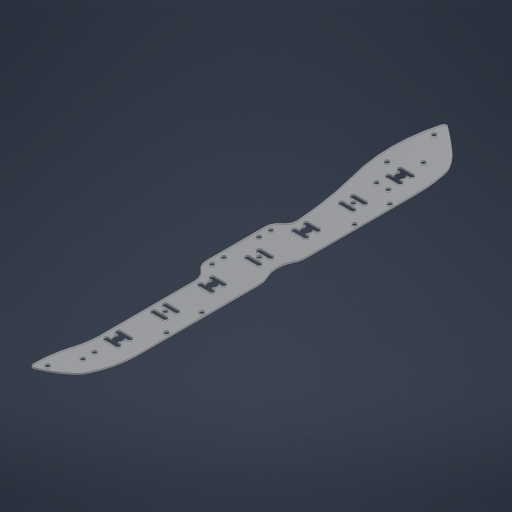
# Autodesk Inventor part: sled2
Saved by Autodesk Inventor 2024 (Build 280153000, 153)
## iProperties
Created: 2023-10-30
Part Number: sled2
Material: Polycarbonate, Smoke
Document SubType Name: Modeling
Designer: macbook
Density: 1.2 g/cm^3
Appearance: Polycarbonate - Clear(1)
Author: macbook
Autodesk Inventor part; units mm, degrees
ref_plane "YZ Plane" through (0, 0, 0) normal (1, 0, 0) x (0, 1, 0)
ref_plane "XZ Plane" through (0, 0, 0) normal (0, 1, 0) x (-1, 0, 0)
ref_plane "XY Plane" through (0, 0, 0) normal (0, 0, 1) x (1, 0, 0)
sketch "Sketch2" plane through (0, 0, 0) normal (0, 1, 0) x (-1, 0, 0)
  line L0 (25.3485, -88.9331) -> (25.3485, -76.2331)
  line L1 (25.3485, -76.2331) -> (0.0063, -76.2331)
  line L2 (0.0063, -76.2331) -> (0.0055, -63.5331)
  line L3 (0.1328, -20.6833) -> (0.1265, -35.8822)
  line L4 (38.2012, -93.5899) -> (38.2012, -99.9399)
  line L5 (12.8495, -23.9499) -> (19.1995, -23.9501)
  line L6 (19.1995, -23.9501) -> (6.4995, -23.9497)
  line L7 (25.3485, -88.9331) -> (31.6373, -88.0533)
  arc A0 (30.6963, -113.4359) -> (33.2246, -115.3327) centre (248.7957, 174.6442) ccw
  line L8 (38.2825, -88.8911) -> (38.2774, -69.8411)
  line L9 (38.2774, -69.8411) -> (44.78, -69.8393)
  arc A1 (38.3114, -113.5855) -> (38.3007, -17.4758) centre (-135.3855, -65.5498) ccw
  arc A2 (33.2246, -115.3327) -> (38.3114, -113.5855) centre (35.1695, -112.7166) ccw
  arc A3 (44.8311, -65.5299) -> (38.2642, -32.0968) centre (-43.6087, -65.5397) ccw
  line L10 (6.4995, -23.9497) -> (0.1314, -23.947)
  line L11 (0.1314, -23.947) -> (0.2658, 299.9029) construction
  line L12 (0.2658, 299.9029) -> (25.6658, 299.9029) construction
  line L13 (25.6658, 269.4446) -> (25.6658, -23.6933)
  line L14 (25.6658, -23.6933) -> (39.903, -23.6933)
  line L15 (0.2658, 299.9029) -> (-12.4342, 299.9029)
  line L16 (-12.5436, -23.9601) -> (-12.5436, -35.112)
  arc A4 (-4.3142, -80.5045) -> (7.2064, -94.0414) centre (51.9465, -44.2947) ccw
  arc A5 (-12.5436, -35.112) -> (-9.0134, -68.7415) centre (149.4014, -35.112) ccw
  arc A6 (-5.9833, -77.5413) -> (-4.3142, -80.5045) centre (19.9766, -64.8707) ccw
  arc A7 (-9.0134, -68.7415) -> (-5.9833, -77.5413) centre (28.2561, -60.8297) ccw
  arc A8 (7.2064, -94.0414) -> (30.6963, -113.4359) centre (248.7971, 174.6431) ccw
  line L17 (0.2658, 299.9029) -> (0.1867, 109.403) construction
  line L18 (0.1867, 109.403) -> (-36.5163, 109.4182)
  arc A9 (-9.714, 95.5829) -> (-9.702, 123.2303) centre (-36.5163, 109.4182) ccw
  line L19 (-12.5217, 258.1981) -> (-12.5217, 134.8616)
  line L20 (-12.5436, 83.9322) -> (-12.5436, -23.9601)
  arc A10 (-12.5217, 127.6948) -> (-12.5436, 91.1127) centre (-36.5163, 109.4182) ccw construction
  arc A11 (-12.5217, 134.8616) -> (-9.702, 123.2303) centre (12.8783, 134.8616) ccw
  arc A12 (-9.714, 95.5829) -> (-12.5436, 83.9322) centre (12.8564, 83.9322) ccw
  line L21 (25.6658, 299.9029) -> (25.6658, 331.6529)
  line L22 (25.6658, 331.6529) -> (32.0158, 331.6529)
  arc A13 (35.1908, 331.6395) -> (28.8408, 331.6529) centre (32.0158, 331.6529) ccw
  line L23 (0.2658, 299.9029) -> (0.2658, 325.3029)
  line L24 (32.0158, 331.6529) -> (30.6929, 331.6529)
  arc A14 (29.2214, 292.4497) -> (35.1908, 331.6395) centre (-92.7618, 331.0796) ccw
  line L25 (31.9383, 334.827) -> (31.4142, 334.827)
  arc A15 (31.007, 334.6634) -> (4.0007, 318.3551) centre (65.1249, 247.6497) ccw
  arc A16 (-10.3215, 302.8155) -> (-14.0041, 295.5815) centre (10.1821, 287.8234) ccw
  line L26 (-12.5217, 258.1981) -> (-12.5217, 338.0406)
  arc A17 (-2.1991, 310.3119) -> (-12.5217, 265.7661) centre (88.7553, 265.7661) ccw
  arc A18 (4.0007, 318.3551) -> (-2.1991, 310.3119) centre (20.612, 299.1399) ccw
  line L27 (0.2658, 299.9029) -> (0.2605, 287.2029)
  line L28 (0.2605, 287.2029) -> (12.9605, 287.1977)
  line L29 (0.1867, 109.403) -> (0.221, 191.953)
  line L30 (0.221, 191.953) -> (-7.7165, 191.9562)
  line L31 (0.1867, 109.403) -> (0.1525, 26.853)
  line L32 (0.1525, 26.853) -> (-7.785, 26.853)
  line L33 (-7.785, 26.853) -> (-7.785, -11.247)
  line L34 (-7.7165, 191.9562) -> (-7.7165, 230.0562)
  arc A19 (25.6658, 282.6329) -> (27.2405, 286.6766) centre (-92.7618, 331.0796) ccw
  arc A20 (29.2214, 292.4497) -> (25.6658, 269.4446) centre (101.8658, 269.4446) ccw
  line L35 (25.6658, 109.403) -> (32.0158, 109.403)
  line L36 (32.0158, 109.403) -> (32.0158, 90.353)
  line L37 (32.0158, 90.353) -> (32.0158, 77.653)
  line L38 (32.0158, 109.403) -> (32.0158, 128.453)
  line L39 (32.0158, 128.453) -> (32.0158, 141.153)
  line L40 (32.0158, 109.403) -> (38.3658, 109.403)
  line L41 (38.3658, 109.403) -> (38.3658, 141.153)
  arc A21 (38.3658, 141.153) -> (32.0778, 153.6114) centre (22.8798, 141.153) ccw
  arc A22 (25.6658, 83.9658) -> (25.6658, 78.268) centre (416.3302, 81.1169) ccw
  arc A23 (26.6118, 53.7976) -> (38.3007, -17.4758) centre (416.3302, 81.1169) ccw
  arc A24 (25.6658, 166.3155) -> (32.0778, 153.6114) centre (41.457, 166.3155) ccw
  line L42 (38.3658, 109.403) -> (38.3658, 77.653)
  arc A25 (32.0778, 65.1945) -> (38.3658, 77.653) centre (22.8798, 77.653) ccw
  arc A26 (32.0778, 65.1945) -> (30.3394, 63.7048) centre (41.457, 52.4904) ccw
  arc A27 (30.3394, 63.7048) -> (26.6118, 53.7976) centre (39.2807, 54.6857) ccw
  line L43 (25.6658, 299.9029) -> (25.6658, 325.3029)
  line L44 (12.9605, 287.1977) -> (12.9605, 299.8977)
  point P0 (0.0775, -39.6857)
  point P1 (12.8012, -68.1967)
  point P2 (37.0807, -118.1599)
  point P3 (33.0954, -49.1463)
  point P4 (33.0954, -99.9463)
  point P5 (33.0954, -99.9463)
  point P6 (33.0954, -49.1463)
  point P7 (30.6993, 334.5421)
  point P8 (25.6658, 160.9899)
  point P9 (25.6658, 57.8161)
  point P10 (25.6658, 52.4904)
  point P11 (26.3876, 57.21)
  dimension "d3" = 12.7
  dimension "d5" = 12.7
  dimension "d37" = 6.35
  dimension "d54" = 6.35
  dimension "d55" = 25.4
  dimension "d58" = 19.05
  dimension "d82" = 323.85
  dimension "d83" = 25.4
  dimension "d84" = 12.7
  dimension "d85" = 38.1
  dimension "d86" = 190.5
  dimension "d87" = 60.325
  dimension "d88" = 36.703
  dimension "d89" = 25.4
  dimension "d93" = 6.35
  dimension "d94" = 6.35
  dimension "d95" = 31.75
  dimension "d97" = 25.4
  dimension "d99" = 25.4
  dimension "d102" = 25.4
  dimension "d103" = 12.7
  dimension "d104" = 12.7
  dimension "d105" = 82.55
  dimension "d106" = 7.9375
  dimension "d107" = 82.55
  dimension "d108" = 38.1
  dimension "d109" = 38.1
  dimension "d110" = 76.2
  dimension "d111" = 6.35
  dimension "d112" = 19.05
  dimension "d113" = 12.7
  dimension "d114" = 19.05
  dimension "d115" = 12.7
  dimension "d116" = 6.35
  dimension "d117" = 31.75
  dimension "d118" = 12.7
  dimension "d119" = 12.7
  constraints: 90 end point, 67 point on circle, 28 centre point, 22 tangent, 21 point on line, 18 coincident, 13 perpendicular, 10 vertical, 6 horizontal, 5 symmetric about line, 1 equal radius, 1 midpoint, 2 other
  measures "d3" distance of L0.start L0.end
  measures "d5" distance of L1.end L2.end
  measures "d37" distance of L5.start L5.end
  measures "d54" distance of L0.start L7.end
  measures "d55" distance of L7.end A0.start
  measures "d58" distance of L8.start L8.end
  measures "d82" distance of L10.end L11.end
  measures "d83" distance of L11.end L12.end
  measures "d84" distance of L11.end L15.end
  measures "d85" radius of A7
  measures "d86" distance of L11.end L17.end
  measures "d87" diameter of A9
  measures "d88" distance of L17.end L18.end
  measures "d89" radius of A11
  measures "d93" distance of L21.end L22.end
  measures "d94" diameter of A13
  measures "d95" distance of L12.end L21.end
  measures "d97" distance of L11.end L23.end
  measures "d99" radius of A16
  measures "d102" radius of A18
  measures "d103" distance of L11.end L27.end
  measures "d104" distance of L27.end L28.end
  measures "d105" distance of L17.end L29.end
  measures "d106" distance of L29.end L30.end
  measures "d107" distance of L17.end L31.end
  measures "d108" distance of L33.start L33.end
  measures "d109" distance of L34.start L34.end
  measures "d110" radius of A20
  measures "d111" distance of L35.start L35.end
  measures "d112" distance of L35.end L36.end
  measures "d113" distance of L36.end L37.end
  measures "d114" distance of L35.end L38.end
  measures "d115" distance of L38.end L39.end
  measures "d116" distance of L40.start L40.end
  measures "d117" distance of L40.end L41.end
  measures "d118" radius of A27
  measures "d119" distance of L44.start L44.end
extrude "Extrusion1" add sketch "Sketch2" along normal blind 1.5875 contours A8 A4 A6 A7 A5 L16 L20 A12 A9 A11 L19 L26 A17 L15 L23 A18 A15 A13 A14 A20 L13 A22 L14 A1 A2 A0 | L14 L13 L35 L40 L42 A25 A26 A27 A23 A1 | A22 L13 | L13 A24 A21 L41 L40 L35 | A17 A18 L23 L15 | A15 A13
hole "Hole3" at (-6.4995, 0, -23.9497) at (-19.1995, 0, -23.9501) at (-12.8012, 0, -68.1967) at (-33.0954, 0, -49.1463) at (-33.0954, 0, -99.9463) at (-12.9605, 0, 287.1977) at (7.7165, 0, 191.9562) at (7.785, 0, 26.853) at (7.785, 0, -11.247) at (7.7165, 0, 230.0562) at (-32.0158, 0, 141.153) at (-32.0158, 0, 128.453) at (-32.0158, 0, 90.353) at (-32.0158, 0, 77.653) at (-25.6658, 0, 325.3029) at (-12.9605, 0, 299.8977) direction (0, 1, 0) diameter 4.7625 end through all
sketch "Sketch4" plane through (0, 1.5875, 0) normal (0, 1, 0) x (1, 0, 0)
  line L0 (-19.1995, 23.9497) -> (-19.1995, 42.9997) construction
  line L1 (-19.1995, 23.9497) -> (-0.1495, 23.9497) construction
  line L2 (-19.1995, 42.9997) -> (-12.8495, 42.9997)
  line L3 (-6.4995, 23.9497) -> (-6.4995, 36.6497) construction
  line L4 (-6.4995, 36.6497) -> (-19.1995, 36.6497) construction
  arc A0 (-19.1995, 39.0309) -> (-19.1995, 34.2684) centre (-19.1995, 36.6497) ccw
  arc A1 (-6.4995, 34.2684) -> (-6.4995, 39.0309) centre (-6.4995, 36.6497) ccw
  line L5 (-19.1995, 34.2684) -> (-6.4995, 34.2684)
  line L6 (-6.4995, 36.6497) -> (-6.4995, 49.3497) construction
  line L7 (-6.4995, 49.3497) -> (-19.1995, 49.3497) construction
  arc A2 (-19.1995, 51.7309) -> (-19.1995, 46.9684) centre (-19.1995, 49.3497) ccw
  arc A3 (-6.4995, 46.9684) -> (-6.4995, 51.7309) centre (-6.4995, 49.3497) ccw
  line L8 (-6.4995, 51.7309) -> (-19.1995, 51.7309)
  line L9 (-12.8495, 34.2684) -> (-12.8495, 36.6497)
  line L10 (-12.8495, 36.6497) -> (-19.1995, 36.6497)
  line L11 (-19.1995, 39.0309) -> (-16.0205, 39.0309)
  line L12 (-6.4995, 39.0309) -> (-9.6785, 39.0309)
  line L13 (-6.4995, 46.9684) -> (-9.2483, 46.9684)
  line L14 (-19.1995, 46.9684) -> (-16.4508, 46.9684)
  arc A4 (-9.8454, 39.5008) -> (-9.4379, 46.5192) centre (-12.8495, 43.1963) ccw
  arc A5 (-16.2612, 46.5192) -> (-15.8536, 39.5008) centre (-12.8495, 43.1963) ccw
  arc A6 (-9.8454, 39.5008) -> (-9.6785, 39.0309) centre (-9.6785, 39.2955) ccw
  arc A7 (-16.0205, 39.0309) -> (-15.8536, 39.5008) centre (-16.0205, 39.2955) ccw
  arc A8 (-16.2612, 46.5192) -> (-16.4508, 46.9684) centre (-16.4508, 46.7038) ccw
  arc A9 (-9.2483, 46.9684) -> (-9.4379, 46.5192) centre (-9.2483, 46.7038) ccw
  line L15 (-6.4995, 23.9497) -> (-12.8495, 23.9497) construction
  line L16 (-12.8495, 23.9497) -> (-12.8495, -77.6503) construction
  line L17 (-12.8495, -77.6503) -> (-12.8495, -179.2503) construction
  line L18 (-12.8495, -179.2503) -> (-12.8495, -280.8503) construction
  arc A10 (-19.1995, -49.8691) -> (-19.1995, -54.6316) centre (-19.1995, -52.2503) ccw
  arc A11 (-6.4995, -67.3316) -> (-6.4995, -62.5691) centre (-6.4995, -64.9503) ccw
  arc A12 (-6.4995, -54.6316) -> (-6.4995, -49.8691) centre (-6.4995, -52.2503) ccw
  line L19 (-6.4995, -54.6316) -> (-9.2483, -54.6316)
  line L20 (-19.1995, -54.6316) -> (-16.4508, -54.6316)
  arc A13 (-16.2612, -55.0808) -> (-16.4508, -54.6316) centre (-16.4508, -54.8962) ccw
  line L21 (-19.1995, -58.6003) -> (-12.8495, -58.6003)
  line L22 (-6.4995, -49.8691) -> (-19.1995, -49.8691)
  arc A14 (-9.2483, -54.6316) -> (-9.4379, -55.0808) centre (-9.2483, -54.8962) ccw
  arc A15 (-16.2612, -55.0808) -> (-15.8536, -62.0992) centre (-12.8495, -58.4037) ccw
  line L23 (-6.4995, -52.2503) -> (-19.1995, -52.2503) construction
  arc A16 (-9.8454, -62.0992) -> (-9.4379, -55.0808) centre (-12.8495, -58.4037) ccw
  line L24 (-6.4995, -64.9503) -> (-6.4995, -52.2503) construction
  arc A17 (-19.1995, -62.5691) -> (-19.1995, -67.3316) centre (-19.1995, -64.9503) ccw
  line L25 (-6.4995, -64.9503) -> (-19.1995, -64.9503) construction
  line L26 (-19.1995, -67.3316) -> (-6.4995, -67.3316)
  line L27 (-19.1995, -62.5691) -> (-16.0205, -62.5691)
  arc A18 (-16.0205, -62.5691) -> (-15.8536, -62.0992) centre (-16.0205, -62.3045) ccw
  line L28 (-12.8495, -64.9503) -> (-19.1995, -64.9503)
  arc A19 (-9.8454, -62.0992) -> (-9.6785, -62.5691) centre (-9.6785, -62.3045) ccw
  line L29 (-6.4995, -62.5691) -> (-9.6785, -62.5691)
  line L30 (-12.8495, -67.3316) -> (-12.8495, -64.9503)
  arc A20 (-19.1995, -151.4691) -> (-19.1995, -156.2316) centre (-19.1995, -153.8503) ccw
  arc A21 (-6.4995, -168.9316) -> (-6.4995, -164.1691) centre (-6.4995, -166.5503) ccw
  arc A22 (-6.4995, -156.2316) -> (-6.4995, -151.4691) centre (-6.4995, -153.8503) ccw
  line L31 (-6.4995, -156.2316) -> (-9.2483, -156.2316)
  line L32 (-19.1995, -156.2316) -> (-16.4508, -156.2316)
  arc A23 (-16.2612, -156.6808) -> (-16.4508, -156.2316) centre (-16.4508, -156.4962) ccw
  line L33 (-19.1995, -160.2003) -> (-12.8495, -160.2003)
  line L34 (-6.4995, -151.4691) -> (-19.1995, -151.4691)
  arc A24 (-9.2483, -156.2316) -> (-9.4379, -156.6808) centre (-9.2483, -156.4962) ccw
  arc A25 (-16.2612, -156.6808) -> (-15.8536, -163.6992) centre (-12.8495, -160.0037) ccw
  line L35 (-6.4995, -153.8503) -> (-19.1995, -153.8503) construction
  arc A26 (-9.8454, -163.6992) -> (-9.4379, -156.6808) centre (-12.8495, -160.0037) ccw
  line L36 (-6.4995, -166.5503) -> (-6.4995, -153.8503) construction
  arc A27 (-19.1995, -164.1691) -> (-19.1995, -168.9316) centre (-19.1995, -166.5503) ccw
  line L37 (-6.4995, -166.5503) -> (-19.1995, -166.5503) construction
  line L38 (-19.1995, -168.9316) -> (-6.4995, -168.9316)
  line L39 (-19.1995, -164.1691) -> (-16.0205, -164.1691)
  arc A28 (-16.0205, -164.1691) -> (-15.8536, -163.6992) centre (-16.0205, -163.9045) ccw
  line L40 (-12.8495, -166.5503) -> (-19.1995, -166.5503)
  arc A29 (-9.8454, -163.6992) -> (-9.6785, -164.1691) centre (-9.6785, -163.9045) ccw
  line L41 (-6.4995, -164.1691) -> (-9.6785, -164.1691)
  line L42 (-12.8495, -168.9316) -> (-12.8495, -166.5503)
  arc A30 (-19.1995, -253.0691) -> (-19.1995, -257.8316) centre (-19.1995, -255.4503) ccw
  arc A31 (-6.4995, -270.5316) -> (-6.4995, -265.7691) centre (-6.4995, -268.1503) ccw
  arc A32 (-6.4995, -257.8316) -> (-6.4995, -253.0691) centre (-6.4995, -255.4503) ccw
  line L43 (-6.4995, -257.8316) -> (-9.2483, -257.8316)
  line L44 (-19.1995, -257.8316) -> (-16.4508, -257.8316)
  arc A33 (-16.2612, -258.2808) -> (-16.4508, -257.8316) centre (-16.4508, -258.0962) ccw
  line L45 (-19.1995, -261.8003) -> (-12.8495, -261.8003)
  line L46 (-6.4995, -253.0691) -> (-19.1995, -253.0691)
  arc A34 (-9.2483, -257.8316) -> (-9.4379, -258.2808) centre (-9.2483, -258.0962) ccw
  arc A35 (-16.2612, -258.2808) -> (-15.8536, -265.2992) centre (-12.8495, -261.6037) ccw
  line L47 (-6.4995, -255.4503) -> (-19.1995, -255.4503) construction
  arc A36 (-9.8454, -265.2992) -> (-9.4379, -258.2808) centre (-12.8495, -261.6037) ccw
  line L48 (-6.4995, -268.1503) -> (-6.4995, -255.4503) construction
  arc A37 (-19.1995, -265.7691) -> (-19.1995, -270.5316) centre (-19.1995, -268.1503) ccw
  line L49 (-6.4995, -268.1503) -> (-19.1995, -268.1503) construction
  line L50 (-19.1995, -270.5316) -> (-6.4995, -270.5316)
  line L51 (-19.1995, -265.7691) -> (-16.0205, -265.7691)
  arc A38 (-16.0205, -265.7691) -> (-15.8536, -265.2992) centre (-16.0205, -265.5045) ccw
  line L52 (-12.8495, -268.1503) -> (-19.1995, -268.1503)
  arc A39 (-9.8454, -265.2992) -> (-9.6785, -265.7691) centre (-9.6785, -265.5045) ccw
  line L53 (-6.4995, -265.7691) -> (-9.6785, -265.7691)
  line L54 (-12.8495, -270.5316) -> (-12.8495, -268.1503)
  line L55 (-12.8495, 23.9497) -> (-12.8495, -26.8503) construction
  arc A40 (-19.1995, 0.9309) -> (-19.1995, -3.8316) centre (-19.1995, -1.4503) ccw
  arc A41 (-6.4995, -16.5316) -> (-6.4995, -11.7691) centre (-6.4995, -14.1503) ccw
  arc A42 (-6.4995, -3.8316) -> (-6.4995, 0.9309) centre (-6.4995, -1.4503) ccw
  line L56 (-6.4995, -3.8316) -> (-9.2483, -3.8316)
  line L57 (-19.1995, -3.8316) -> (-16.4508, -3.8316)
  line L58 (-6.4995, 0.9309) -> (-19.1995, 0.9309)
  line L59 (-6.4995, -1.4503) -> (-19.1995, -1.4503) construction
  line L60 (-6.4995, -14.1503) -> (-6.4995, -1.4503) construction
  arc A43 (-19.1995, -11.7691) -> (-19.1995, -16.5316) centre (-19.1995, -14.1503) ccw
  line L61 (-6.4995, -14.1503) -> (-19.1995, -14.1503) construction
  line L62 (-19.1995, -16.5316) -> (-6.4995, -16.5316)
  line L63 (-19.1995, -11.7691) -> (-16.0205, -11.7691)
  line L64 (-12.8495, -14.1503) -> (-19.1995, -14.1503)
  line L65 (-6.4995, -11.7691) -> (-9.6785, -11.7691)
  line L66 (-12.8495, -16.5316) -> (-12.8495, -14.1503)
  circle A44 centre (-12.8495, -7.6037) radius 2.3812
  line L67 (-16.0205, -11.7691) -> (-9.6785, -11.7691)
  line L68 (-16.4508, -3.8316) -> (-9.2483, -3.8316)
  line L69 (-12.8495, -77.6503) -> (-12.8495, -128.4503)
  line L70 (-6.4995, -115.7503) -> (-6.4995, -103.0503) construction
  line L71 (-6.4995, -115.7503) -> (-19.1995, -115.7503) construction
  line L72 (-6.4995, -113.3691) -> (-9.6785, -113.3691)
  line L73 (-19.1995, -105.4316) -> (-16.4508, -105.4316)
  line L74 (-6.4995, -103.0503) -> (-19.1995, -103.0503) construction
  line L75 (-6.4995, -100.6691) -> (-19.1995, -100.6691)
  arc A45 (-19.1995, -100.6691) -> (-19.1995, -105.4316) centre (-19.1995, -103.0503) ccw
  line L76 (-12.8495, -115.7503) -> (-19.1995, -115.7503)
  line L77 (-19.1995, -113.3691) -> (-16.0205, -113.3691)
  line L78 (-6.4995, -105.4316) -> (-9.2483, -105.4316)
  arc A46 (-6.4995, -105.4316) -> (-6.4995, -100.6691) centre (-6.4995, -103.0503) ccw
  arc A47 (-6.4995, -118.1316) -> (-6.4995, -113.3691) centre (-6.4995, -115.7503) ccw
  arc A48 (-19.1995, -113.3691) -> (-19.1995, -118.1316) centre (-19.1995, -115.7503) ccw
  line L79 (-12.8495, -118.1316) -> (-12.8495, -115.7503)
  line L80 (-19.1995, -118.1316) -> (-6.4995, -118.1316)
  circle A49 centre (-12.8495, -109.2037) radius 2.3812
  line L81 (-16.0205, -113.3691) -> (-9.6785, -113.3691)
  line L82 (-16.4508, -105.4316) -> (-9.2483, -105.4316)
  line L83 (-12.8495, -179.2503) -> (-12.8495, -230.0503)
  arc A50 (-19.1995, -202.2691) -> (-19.1995, -207.0316) centre (-19.1995, -204.6503) ccw
  line L84 (-12.8495, -219.7316) -> (-12.8495, -217.3503)
  line L85 (-12.8495, -217.3503) -> (-19.1995, -217.3503)
  arc A51 (-19.1995, -214.9691) -> (-19.1995, -219.7316) centre (-19.1995, -217.3503) ccw
  line L86 (-6.4995, -217.3503) -> (-6.4995, -204.6503) construction
  circle A52 centre (-12.8495, -210.8037) radius 2.3812
  line L87 (-19.1995, -207.0316) -> (-16.4508, -207.0316)
  line L88 (-16.4508, -207.0316) -> (-9.2483, -207.0316)
  line L89 (-6.4995, -204.6503) -> (-19.1995, -204.6503) construction
  line L90 (-6.4995, -202.2691) -> (-19.1995, -202.2691)
  line L91 (-6.4995, -207.0316) -> (-9.2483, -207.0316)
  arc A53 (-6.4995, -207.0316) -> (-6.4995, -202.2691) centre (-6.4995, -204.6503) ccw
  line L92 (-6.4995, -214.9691) -> (-9.6785, -214.9691)
  arc A54 (-6.4995, -219.7316) -> (-6.4995, -214.9691) centre (-6.4995, -217.3503) ccw
  line L93 (-16.0205, -214.9691) -> (-9.6785, -214.9691)
  line L94 (-19.1995, -214.9691) -> (-16.0205, -214.9691)
  line L95 (-19.1995, -219.7316) -> (-6.4995, -219.7316)
  line L96 (-6.4995, -217.3503) -> (-19.1995, -217.3503) construction
  point P0 (0, 0)
  point P1 (-15.1584, 39.0309)
  point P2 (-10.5407, 39.0309)
  point P3 (-9.9422, 46.9684)
  point P4 (-15.7569, 46.9684)
  point P5 (-15.7569, -54.6316)
  point P6 (-9.9422, -54.6316)
  point P7 (-15.1584, -62.5691)
  point P8 (-10.5407, -62.5691)
  point P9 (-15.7569, -156.2316)
  point P10 (-9.9422, -156.2316)
  point P11 (-15.1584, -164.1691)
  point P12 (-10.5407, -164.1691)
  point P13 (-15.7569, -257.8316)
  point P14 (-9.9422, -257.8316)
  point P15 (-15.1584, -265.7691)
  point P16 (-10.5407, -265.7691)
  point P17 (-15.7569, -3.8316)
  point P18 (-9.9422, -3.8316)
  point P19 (-15.1584, -11.7691)
  point P20 (-10.5407, -11.7691)
  point P21 (-10.5407, -113.3691)
  point P22 (-15.1584, -113.3691)
  point P23 (-15.7569, -105.4316)
  point P24 (-9.9422, -105.4316)
  point P25 (-15.7569, -207.0316)
  point P26 (-9.9422, -207.0316)
  point P27 (-10.5407, -214.9691)
  point P28 (-15.1584, -214.9691)
  dimension "d121" = 19.05
  dimension "d122" = 90
  dimension "d123" = 6.35
  dimension "d124" = 12.7
  dimension "d125" = 6.35
  dimension "d126" = 0.2646
  dimension "d129" = 101.6
  dimension "d130" = 101.6
  dimension "d131" = 101.6
  dimension "d132" = 6.35
  dimension "d133" = 6.35
  dimension "d134" = 0.2646
  dimension "d135" = 6.35
  dimension "d136" = 6.35
  dimension "d137" = 0.2646
  dimension "d138" = 6.35
  dimension "d139" = 6.35
  dimension "d140" = 0.2646
  dimension "d141" = 50.8
  dimension "d143" = 6.35
  dimension "d145" = 4.7625
  dimension "d146" = 50.8
  dimension "d148" = 6.35
  dimension "d149" = 4.7625
  dimension "d152" = 50.8
  dimension "d153" = 6.35
  dimension "d154" = 4.7625
  constraints: 194 end point, 120 point on circle, 55 centre point, 55 point on line, 46 tangent, 28 coincident, 17 midpoint, 13 collinear, 12 equal radius, 11 perpendicular, 10 vertical, 8 horizontal, 7 parallel
  measures "d121" distance of L0.start L2.start
  measures "d122" angle of L1 L0
  measures "d123" distance of L2.start L2.end
  measures "d124" distance of L3.start L4.start
  measures "d125" distance of L10.start L10.end
  measures "d126" radius of A6
  measures "d129" distance of L15.end L16.end
  measures "d130" distance of L16.end L17.end
  measures "d131" distance of L17.end L18.end
  measures "d132" distance of L21.start L21.end
  measures "d133" distance of L28.start L28.end
  measures "d134" radius of A19
  measures "d135" distance of L33.start L33.end
  measures "d136" distance of L40.start L40.end
  measures "d137" radius of A29
  measures "d138" distance of L45.start L45.end
  measures "d139" distance of L52.start L52.end
  measures "d140" radius of A39
  measures "d141" distance of L15.end L55.end
  measures "d143" distance of L64.start L64.end
  measures "d145" diameter of A44
  measures "d146" distance of L16.end L69.end
  measures "d148" distance of L79.end L76.end
  measures "d149" diameter of A49
  measures "d152" distance of L17.end L83.end
  measures "d153" distance of L84.end L85.end
  measures "d154" diameter of A52
extrude "Extrusion3" cut sketch "Sketch4" against normal blind 25.4
body "Solid1"
